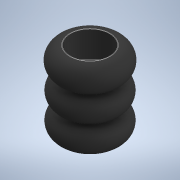
# Autodesk Inventor part: Air Suspension Air Bag
Saved by Autodesk Inventor 2022 (Build 260153000, 153)
## iProperties
Created: 2021-07-29
Part Number: Air Suspension Air Bag
Material: Rubber, Silicone
Document SubType Name: Modeling
Designer: WASHINGTON
Density: 1.25 g/cm^3
Appearance: Rubber - Black
Author: WASHINGTON
Autodesk Inventor part; units mm, degrees
ref_plane "YZ Plane" through (0, 0, 0) normal (1, 0, 0) x (0, 1, 0)
ref_plane "XZ Plane" through (0, 0, 0) normal (0, 1, 0) x (-1, 0, 0)
ref_plane "XY Plane" through (0, 0, 0) normal (0, 0, 1) x (1, 0, 0)
sketch "Sketch2" plane through (0, 0, 0) normal (0, 0, 1) x (1, 0, 0)
  point P0 (0, 0)
sketch "Sketch3" plane through (0, 0, 0) normal (0, 0, 1) x (1, 0, 0)
  line L0 (0, 0) -> (25, 0)
  line L1 (25, 50) -> (0, 50)
  line L2 (0, 50) -> (0, 0)
  line L3 (0, 16.6667) -> (12.5, 16.6667)
  line L4 (0, 33.3334) -> (12.8745, 33.3334)
  arc A0 (12.5, 33.3334) -> (12.5, 50) centre (12.6873, 41.6667) ccw
  arc A1 (12.5, 16.6667) -> (12.5, 33.3334) centre (12.3127, 25.0001) ccw
  arc A2 (12.5, 0) -> (12.5, 16.6667) centre (12.3362, 8.3334) ccw
  point P0 (12.8745, 50)
  dimension "d2" = 25
  constraints: 10 end point, 7 point on circle, 3 centre point, 3 point on line, 2 midpoint, 1 horizontal, 1 parallel, 1 tangent
  measures "d2" distance of L1.end L1.start
revolve "Revolution1" add sketch "Sketch3" angle 360 about axis through (0, 50, 0) along (0, -1, 0)
sketch "Sketch4" plane through (0, 50, 0) normal (0, 1, 0) x (1, 0, 0)
  circle A0 centre (0, 0) radius 12.5
  constraints: 1 centre point, 1 coincident
extrude "Extrusion1" cut sketch "Sketch4" against normal through all
body "Solid1"
